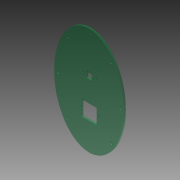
# Autodesk Inventor part: TopCover
Saved by Autodesk Inventor 2015 (Build 190159000, 159)
## iProperties
Created: 2015-10-10
Part Number: TopCover
Material: Generic
Document SubType Name: Modeling
Designer: styku
Density: 1 g/cm^3
Appearance: Clear - Green 1
Mass: 67.6531 g
Surface Area: 483.612 cm^2
Volume: 67.6531 cm^3
Author: styku
Autodesk Inventor part; units mm, degrees
ref_plane "YZ Plane" through (0, 0, 0) normal (1, 0, 0) x (0, 1, 0)
ref_plane "XZ Plane" through (0, 0, 0) normal (0, 1, 0) x (-1, 0, 0)
ref_plane "XY Plane" through (0, 0, 0) normal (0, 0, 1) x (1, 0, 0)
sketch "Sketch1" plane through (0, 0, 0) normal (0, 1, 0) x (-1, 0, 0)
  circle A0 centre (50, 0) radius 1.75
  circle A1 centre (35.016, -56.1406) radius 1.75
  line L0 (0, 113.2764) -> (0, -120.1992) construction
  line L1 (64.7812, 0) -> (-65.3256, 0) construction
  ellipse E0 centre (0, 0) end of major axis (-50, 0) minor radius 78.647 construction
  circle A2 centre (-50, 0) radius 1.75
  circle A3 centre (-35.016, -56.1406) radius 1.75
  circle A4 centre (35.016, 56.1406) radius 1.75
  circle A5 centre (-35.016, 56.1406) radius 1.75
  ellipse E1 centre (0, 0) end of major axis (-0.2534, -85.9996) minor radius 56
  circle A6 centre (10.5, 32.5) radius 1
  circle A7 centre (10.5, 20) radius 1
  circle A8 centre (-10.5, 32.5) radius 1
  circle A9 centre (-10.5, 20) radius 1
  circle A10 centre (14, -30) radius 1
  circle A11 centre (-14, -30) radius 1
  line L2 (12, -18) -> (-12, -18)
  line L3 (-12, -18) -> (-12, -42)
  line L4 (-12, -42) -> (12, -42)
  line L5 (12, -42) -> (12, -18)
  line L6 (-4.25, 24.25) -> (4.25, 24.25)
  line L7 (4.25, 24.25) -> (4.25, 15.75)
  line L8 (4.25, 15.75) -> (-4.25, 15.75)
  line L9 (-4.25, 15.75) -> (-4.25, 24.25)
  dimension "d55" = 78.647
  dimension "d56" = 50
  dimension "d60" = 86
  dimension "d61" = 56
  dimension "d49" = 3.5
  dimension "d58" = 3.5
  dimension "d59" = 35.016
  dimension "d66" = 2
  dimension "d69" = 12.5
  dimension "d72" = 21
  dimension "d75" = 10.5
  dimension "d76" = 20
  dimension "d77" = 2
  dimension "d78" = 28
  dimension "d79" = 30
  dimension "d80" = 24
  dimension "d81" = 24
  dimension "d82" = 12
  dimension "d83" = 12
  dimension "d84" = 8.5
  dimension "d85" = 8.5
  dimension "d86" = 4.25
  dimension "d87" = 4.25
  constraints: 20 end point, 12 centre point, 6 horizontal, 5 symmetric about line, 4 parallel, 3 vertical, 2 coincident, 2 perpendicular, 1 point on line, 17 other
  measures "d49" diameter of A1
  measures "d58" diameter of A0
  measures "d59" distance from line of L0 A1.centre
  measures "d66" diameter of A6
  measures "d69" distance of A6.centre A7.centre
  measures "d72" distance of A6.centre A8.centre
  measures "d75" distance from line of L0 A6.centre
  measures "d76" distance from line of L1 A7.centre
  measures "d77" diameter of A10
  measures "d78" distance of A11.centre A10.centre
  measures "d79" distance from line of L1 A11.centre
  measures "d80" distance of L4.end L3.end
  measures "d81" distance of L2.end L3.end
  measures "d82" distance between parallel lines of L0 L5
  measures "d83" distance from line of A11.centre L2
  measures "d84" distance of L7.end L8.end
  measures "d85" distance of L6.end L7.end
  measures "d86" distance between parallel lines of L0 L7
  measures "d87" distance from line of A9.centre L6
extrude "Extrusion7" add sketch "Sketch1" along normal blind 3
body "Solid4"
